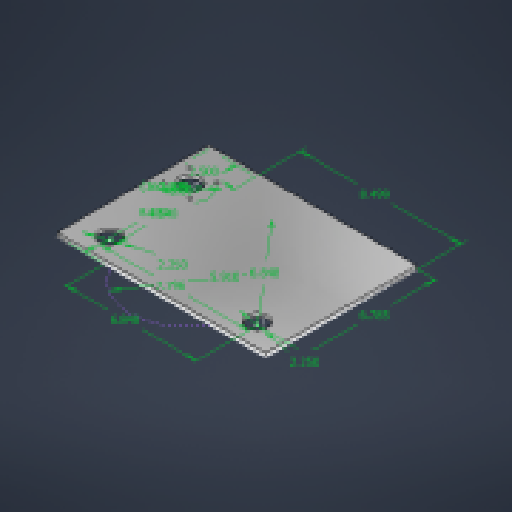
# Autodesk Inventor part: PLATE,KICKER,OUTSIDE
Saved by Autodesk Inventor 2026 (Build 300175000, 175)
## iProperties
Created: 2026-02-07
Part Number: PLATE,KICKER,OUTSIDE
Material: Aluminum 6061
Document SubType Name: Sheet Metal
Designer: littl
Density: 2.7 g/cm^3
Appearance: Aluminum - Flat
Sheet Metal Rule: Default
Author: littl
Autodesk Inventor part; units mm, degrees
ref_plane "YZ Plane" through (0, 0, 0) normal (1, 0, 0) x (0, 1, 0)
ref_plane "XZ Plane" through (0, 0, 0) normal (0, 1, 0) x (-1, 0, 0)
ref_plane "XY Plane" through (0, 0, 0) normal (0, 0, 1) x (1, 0, 0)
sketch "Sketch1" plane through (0, 0, 0) normal (0, 1, 0) x (-1, 0, 0)
  line L0 (-107.95, 101.6) -> (107.95, 101.6)
  line L1 (107.95, 101.6) -> (107.95, -101.6) construction
  line L2 (107.95, -101.6) -> (-107.95, -101.6)
  line L3 (-107.95, -101.6) -> (-107.95, 101.6)
  line L4 (-107.95, 101.6) -> (107.95, -101.6) construction
  line L5 (107.95, 101.6) -> (-107.95, -101.6) construction
  circle A0 centre (-65.9765, 70.739) radius 28.575 construction
  line L6 (107.95, 101.6) -> (171.45, 101.6)
  line L7 (171.45, 101.6) -> (171.45, -101.6)
  line L8 (171.45, -101.6) -> (107.95, -101.6)
  line L9 (107.95, -101.6) -> (107.95, 101.6) construction
  circle A1 centre (132.0339, 70.739) radius 28.575 construction
  circle A2 centre (139.7, -44.5175) radius 30.1625 construction
  circle A3 centre (32.8287, 67.1746) radius 75.057 construction
  arc A4 (-42.5309, -101.6) -> (105.9516, 44.4492) centre (-65.9765, 70.739) ccw construction
  line L10 (139.7, -25.9224) -> (139.7, -58.8783) construction
  line L11 (157.6605, -26.557) -> (139.7, -44.5175) construction
  point P0 (0, 0)
  point P1 (121.7395, -26.557)
  point P2 (121.7395, -62.478)
  point P3 (157.6605, -62.478)
  dimension "d0" = 203.2
  dimension "d1" = 215.9
  dimension "d5" = 57.15
  dimension "d9" = 57.15
  dimension "d10" = 198.0104
  dimension "d12" = 115.5112
  dimension "d13" = 60.325
  dimension "d14" = 150.114
  dimension "d15" = 172.339
  dimension "d17" = 173.9265
  dimension "d18" = 173.9265
  dimension "d28" = 25.4
  dimension "d31" = 360
  dimension "d33" = 45
  dimension "d79" = 279.4
  constraints: 24 end point, 5 centre point, 4 parallel, 2 coincident, 2 horizontal, 2 midpoint, 2 perpendicular, 2 point on circle, 2 point on line, 1 collinear, 1 horizontal alignment, 1 tangent, 1 vertical, 6 other
  measures "d0" distance of L0.end L1.end
  measures "d1" distance of L1.end L2.end
  measures "d5" diameter of A0
  measures "d9" diameter of A1
  measures "d10" distance of A0.centre A1.centre
  measures "d12" distance of A1.centre point (139.7, -44.518)
  measures "d13" diameter of A2
  measures "d14" diameter of A3
  measures "d15" distance from line of L2 A0.centre
  measures "d17" radius of A4
  measures "d18" distance from line of A0.centre L1
  measures "d28" distance of L11.end L11.start
  measures "d33" angle of L10 L11
  measures "d79" distance between parallel lines of L3 L7
extrude "Plate1" add sketch "Sketch1" along normal blind 4.7625
hole "Hole1" at (65.9765, 0, 70.739) at (-132.0339, 0, 70.739) direction (0, 1, 0) diameter 28.575 depth 4.7625 tip angle 118
sketch "Sketch2" plane through (0, 0, 0) normal (0, -1, 0) x (1, 0, 0)
  circle A0 centre (65.9765, 70.739) radius 14.2875 projected
  point P0 (0, 0)
  point P1 (-73.7235, -62.611)
  point P2 (-32.4485, -91.186)
  point P3 (-99.1235, -14.986)
  dimension "d41" = 165.1
  dimension "d42" = 85.725
  dimension "d43" = 161.925
  dimension "d44" = 98.425
  dimension "d45" = 139.7
  dimension "d46" = 133.35
  measures "d41" horizontal distance of A0.centre point (-99.124, -14.986)
  measures "d42" vertical distance of A0.centre point (-99.124, -14.986)
  measures "d43" vertical distance of A0.centre point (-32.449, -91.186)
  measures "d44" horizontal distance of A0.centre point (-32.449, -91.186)
  measures "d45" horizontal distance of A0.centre point (-73.724, -62.611)
  measures "d46" vertical distance of A0.centre point (-73.724, -62.611)
hole "Hole3" at (-32.4485, 0, -91.186) at (-73.7235, 0, -62.611) at (-99.1235, 0, -14.986) direction (0, 1, 0) diameter 4.9784 depth 4.7625 tip angle 118 clearance for "Flat Head Machine Screw (82)" size "#10" standard "Ansi Unified Screw Threads"
sketch "Sketch3" plane through (0, 0, 0) normal (0, -1, 0) x (1, 0, 0)
  line L0 (107.95, -101.6) -> (-171.45, -101.6) projected
  line L1 (107.95, 101.6) -> (107.95, -101.6) projected
  point P0 (0, 0)
  point P1 (95.25, -76.2)
  point P2 (95.25, -25.4)
  dimension "d54" = 50.8
  dimension "d55" = 25.4
  dimension "d56" = 12.7
  constraints: 1 vertical alignment
  measures "d54" distance of point (95.25, -25.4) point (95.25, -76.2)
  measures "d55" distance from line of L0 point (95.25, -76.2)
  measures "d56" distance from line of L1 point (95.25, -76.2)
hole "Hole4" at (95.25, 0, -76.2) at (95.25, 0, -25.4) direction (0, 1, 0) diameter 4.9784 depth 4.7625 tip angle 118 clearance for "Flat Head Machine Screw (82)" size "#10" standard "Ansi Unified Screw Threads"
sketch "Sketch4" plane through (0, 0, 0) normal (0, -1, 0) x (1, 0, 0)
  line L0 (-171.45, -101.6) -> (-171.45, 101.6) projected
  line L1 (107.95, -101.6) -> (-171.45, -101.6) projected
  line L2 (107.95, 101.6) -> (107.95, -101.6) projected
  point P0 (0, 0)
  point P1 (-158.75, -92.075)
  point P2 (-146.05, -92.075)
  point P3 (-133.35, -92.075)
  point P4 (63.5, -92.075)
  point P5 (50.8, -92.075)
  point P6 (76.2, -92.075)
  dimension "d64" = 12.7
  dimension "d65" = 12.7
  dimension "d66" = 12.7
  dimension "d67" = 9.525
  dimension "d68" = 9.525
  dimension "d69" = 12.7
  dimension "d70" = 12.7
  dimension "d71" = 31.75
  constraints: 4 horizontal alignment
  measures "d64" distance of point (-146.05, -92.075) point (-158.75, -92.075)
  measures "d65" distance of point (-133.35, -92.075) point (-146.05, -92.075)
  measures "d66" distance from line of L0 point (-158.75, -92.075)
  measures "d67" distance from line of L1 point (-158.75, -92.075)
  measures "d68" distance from line of L1 point (50.8, -92.075)
  measures "d69" distance of point (50.8, -92.075) point (63.5, -92.075)
  measures "d70" distance of point (76.2, -92.075) point (63.5, -92.075)
  measures "d71" distance from line of L2 point (76.2, -92.075)
hole "Hole5" at (-158.75, 0, -92.075) at (-146.05, 0, -92.075) at (-133.35, 0, -92.075) at (63.5, 0, -92.075) at (50.8, 0, -92.075) at (76.2, 0, -92.075) direction (0, 1, 0) diameter 4.9784 depth 4.7625 tip angle 118 clearance for "Flat Head Machine Screw (82)" size "#10" standard "Ansi Unified Screw Threads"
fillet "Corner Round1" radius 6.35 4 edges at (-171.45, 2.3813, -101.6) (-171.45, 2.3813, 101.6) (107.95, 2.3813, -101.6) (107.95, 2.3813, 101.6)
sketch "Sketch5" plane through (0, 0, 0) normal (0, -1, 0) x (1, 0, 0)
  circle A0 centre (-132.0339, 70.739) radius 14.2875 projected
  circle A1 centre (-132.0339, 70.739) radius 28.575
  circle A2 centre (65.9765, 70.739) radius 14.2875 projected
  circle A3 centre (65.9765, 70.739) radius 28.575
  line L0 (-165.1, 101.6) -> (101.6, 101.6) projected
  line L1 (-171.45, -95.25) -> (-171.45, 95.25) projected
  line L2 (107.95, 95.25) -> (107.95, -95.25) projected
  point P0 (0, 0)
  point P1 (-165.1, 95.25)
  point P2 (101.6, 95.25)
  point P3 (-50.8, 95.25)
  point P4 (-38.1, 95.25)
  point P5 (-25.4, 95.25)
  dimension "d81" = 57.15
  dimension "d82" = 57.15
  dimension "d83" = 6.35
  dimension "d84" = 6.35
  dimension "d85" = 6.35
  dimension "d86" = 114.3
  dimension "d87" = 12.7
  dimension "d88" = 12.7
  constraints: 4 horizontal alignment, 2 centre point, 2 coincident
  measures "d81" diameter of A1
  measures "d82" diameter of A3
  measures "d83" distance from line of L0 point (-165.1, 95.25)
  measures "d84" distance from line of L1 point (-165.1, 95.25)
  measures "d85" distance from line of L2 point (101.6, 95.25)
  measures "d86" distance of point (-165.1, 95.25) point (-50.8, 95.25)
  measures "d87" distance of point (-38.1, 95.25) point (-50.8, 95.25)
  measures "d88" distance of point (-25.4, 95.25) point (-38.1, 95.25)
hole "Hole6" at (-165.1, 0, 95.25) at (101.6, 0, 95.25) at (-50.8, 0, 95.25) at (-38.1, 0, 95.25) at (-25.4, 0, 95.25) direction (0, 1, 0) diameter 4.9784 depth 4.7625 tip angle 118 clearance for "Flat Head Machine Screw (82)" size "#10" standard "Ansi Unified Screw Threads"
body "Solid1"
